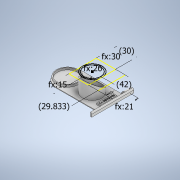
# Autodesk Inventor part: RV
Saved by Autodesk Inventor 2021 (Build 250183000, 183)
## iProperties
Created: 2020-06-05
Part Number: RV
Material: Generic
Document SubType Name: Modeling
Designer: andre
Density: 1 g/cm^3
Appearance: Default
Author: andre
## iProperties of the stored document _3DPrint.ipt
Created: 2020-06-05
Part Number: _3DPrint
Material: Generic
Document SubType Name: Modeling
Designer: andre
Density: 1 g/cm^3
Appearance: Default
Author: andre
Autodesk Inventor part; units mm, degrees
ref_plane "YZ Plane" through (0, 0, 0) normal (1, 0, 0) x (0, 1, 0)
ref_plane "XZ Plane" through (0, 0, 0) normal (0, 1, 0) x (-1, 0, 0)
ref_plane "XY Plane" through (0, 0, 0) normal (0, 0, 1) x (1, 0, 0)
sketch "Sketch1" plane through (0, 0, 0) normal (0, 1, 0) x (-1, 0, 0)
  line L0 (0, 0) -> (85, 0)
  line L1 (85, 0) -> (85, -42)
  line L2 (85, -42) -> (0, -42)
  line L3 (0, -42) -> (0, 0)
  dimension "d0" = 85
  dimension "d1" = 42
  constraints: 8 end point, 2 parallel, 1 horizontal, 1 perpendicular
  measures "d0" distance of L1.end L2.end
  measures "d1" distance of L0.end L1.end
extrude "Extrusion1" add sketch "Sketch1" along normal blind 1
sketch "Sketch2" plane through (0, 1, 0) normal (0, 1, 0) x (1, 0, 0)
  line L0 (-44.8327, 0) -> (-14.8327, 0)
  line L1 (-14.8327, 0) -> (-14.8327, 42)
  line L2 (-14.8327, 42) -> (-44.8327, 42)
  line L3 (-44.8327, 42) -> (-44.8327, 0)
  line L4 (-85, 0) -> (0, 0) projected
  dimension "d4" = 42
  dimension "d5" = 30
  dimension "d6" = 0
  constraints: 8 end point, 2 parallel, 1 horizontal, 1 perpendicular
  measures "d4" distance between parallel lines of L2 L0
  measures "d5" distance between parallel lines of L1 L3
  measures "d6" distance between parallel lines of L4 L0
extrude "Extrusion2" add sketch "Sketch2" along normal blind 28
sketch "Sketch5" plane through (0, 29, 0) normal (0, 1, 0) x (1, 0, 0)
  circle A0 centre (-29.8327, 21) radius 13
  line L0 (-44.8327, 42) -> (-44.8327, 0) projected
  line L1 (-44.8327, 0) -> (-14.8327, 0) projected
  line L2 (-14.8327, 0) -> (-14.8327, 42) projected
  line L3 (-14.8327, 42) -> (-44.8327, 42) projected
  circle A1 centre (-29.8327, 21) radius 15
  line L4 (0, 0) -> (0, 42) projected
  point P0 (-24.115, 0)
  point P1 (-44.8327, 21)
  point P2 (-14.8327, 21)
  point P3 (-19.6709, 0)
  dimension "d20" = 26
  dimension "d21" = 15
  dimension "d22" = 21
  dimension "d23" = 30
  dimension "d24" = 42
  dimension "d34" = 30
  dimension "d63" = 29.8327
  constraints: 2 centre point, 1 coincident
  measures "d20" diameter of A0
  measures "d21" distance from line of L0 A0.centre
  measures "d22" distance from line of L1 A0.centre
  measures "d23" distance between parallel lines of L2 L0
  measures "d24" distance between parallel lines of L3 L1
  measures "d34" diameter of A1
  measures "d63" distance from line of L4 A0.centre
extrude "Extrusion3" cut sketch "Sketch5" against normal blind 28 contours A0
chamfer "Chamfer3" distance 42 distance2 28 1 edges at (-29.8327, 29, -42)
extrude "Extrusion4" cut sketch "Sketch5" against normal blind 28 contours L3 L2 A1 L0 | A1 L2 L1 L0
sketch "Sketch6" plane through (0, 1, 0) normal (0, 1, 0) x (1, 0, 0)
  circle A0 centre (-68, 21) radius 15.75
  line L0 (-85, 0) -> (0, 0) projected
  circle A1 centre (-68, 21) radius 17
  line L1 (-85, 42) -> (-85, 0) projected
  point P0 (-28.5591, 0)
  dimension "d37" = 31.5
  dimension "d38" = 21
  dimension "d39" = 34
  dimension "d64" = 17
  constraints: 2 centre point, 1 coincident
  measures "d37" diameter of A0
  measures "d38" distance from line of L0 A0.centre
  measures "d39" diameter of A1
  measures "d64" distance from line of L1 A1.centre
extrude "Extrusion5" add sketch "Sketch6" along normal blind 3
fillet "Fillet3" radius 21 2 edges at (-85, 0.5, 0) (-85, 0.5, -42)
sketch "Sketch9" plane through (0, 0, 0) normal (1, 0, 0) x (0, 0, -1)
  line L0 (-11.5, 0) -> (53.5, 0)
  line L1 (53.5, 0) -> (53.5, 1)
  line L2 (53.5, 1) -> (-11.5, 1)
  line L3 (-11.5, 1) -> (-11.5, 0)
  line L4 (0, 0) -> (0, 1) projected
  dimension "d49" = 1
  dimension "d50" = 65
  dimension "d53" = 11.5
  constraints: 8 end point, 2 parallel, 1 horizontal, 1 perpendicular
  measures "d49" distance of L1.end L0.end
  measures "d50" distance between parallel lines of L1 L3
  measures "d53" distance between parallel lines of L3 L4
extrude "Extrusion8" add sketch "Sketch9" along normal blind 2
sketch "Sketch10" plane through (0, 1, 0) normal (0, 1, 0) x (1, 0, 0)
  line L0 (0, -11.5) -> (0, 0) projected
  line L1 (2, 53.5) -> (2, -11.5) projected
  line L2 (0, -11.5) -> (2, -11.5)
  line L3 (2, -11.5) -> (2, 53.5)
  line L4 (2, 53.5) -> (0, 53.5)
  line L5 (0, 53.5) -> (0, -11.5)
  point P0 (2, -11.5)
  constraints: 8 end point, 2 parallel, 1 horizontal, 1 perpendicular
extrude "Extrusion9" add sketch "Sketch10" along normal blind 5
sketch "Sketch11" plane through (0, 0, 0) normal (-1, 0, 0) x (0, 0, 1)
  line L0 (11.5, 0) -> (-53.5, 0) projected
  line L1 (-53.5, 6) -> (-42, 6)
  line L2 (-42, 6) -> (-42, 0)
  line L3 (-42, 0) -> (-53.5, 0)
  line L4 (-53.5, 0) -> (-53.5, 6)
  line L5 (-53.5, 6) -> (11.5, 6) projected
  line L6 (-53.5, 0) -> (-53.5, 6) projected
  point P0 (0, 0)
  dimension "d56" = 11.5
  dimension "d58" = 0
  dimension "d65" = 6
  constraints: 8 end point, 2 parallel, 1 horizontal, 1 perpendicular, 1 point on line
  measures "d56" distance of L2.end L3.end
  measures "d58" distance between parallel lines of L6 L4
  measures "d65" distance between parallel lines of L1 L0
extrude "Extrusion10" add sketch "Sketch11" along normal blind 6
fillet "Fillet4" radius 5.9 1 edges at (-6, 6, -47.75)
fillet "Fillet5" radius 2 1 edges at (2, 6, -21)
sketch "Sketch12" plane through (0, 1, 0) normal (0, 1, 0) x (1, 0, 0)
  line L0 (-4.5, 34) -> (-10.3327, 34)
  line L1 (-10.3327, 34) -> (-10.3327, 8)
  line L2 (-10.3327, 8) -> (-4.5, 8)
  line L3 (-4.5, 8) -> (-4.5, 34)
  line L4 (-5.931, 42) -> (-64, 42) projected
  line L5 (-64, 0) -> (0, 0) projected
  line L6 (0, 42) -> (0, -11.5) projected
  circle A0 centre (-29.8327, 21) radius 15 projected
  point P0 (0, 53.5)
  dimension "d66" = 8
  dimension "d67" = 8
  dimension "d68" = 4.5
  dimension "d69" = 4.5
  constraints: 8 end point, 2 parallel, 1 horizontal, 1 perpendicular
  measures "d66" distance between parallel lines of L4 L0
  measures "d67" distance between parallel lines of L5 L2
  measures "d68" distance between parallel lines of L6 L3
  measures "d69" distance edge to line of A0 L1
extrude "Extrusion11" add sketch "Sketch12" along normal blind 2 contours L3 L2 L1 L0
sketch "Sketch13" plane through (0, 3, 0) normal (0, 1, 0) x (1, 0, 0)
  line L0 (-4.5, 34) -> (-4.5, 8) construction
  line L1 (-4.5, 8) -> (-10.3327, 8) construction
  line L2 (-10.3327, 8) -> (-10.3327, 34) construction
  line L3 (-10.3327, 34) -> (-4.5, 34) construction
  line L4 (-4.5, 34) -> (-10.3327, 34) projected
  line L5 (-10.3327, 8) -> (-4.5, 8) projected
  line L6 (-4.5, 8) -> (-4.5, 34) projected
  line L7 (-10.3327, 34) -> (-10.3327, 8) projected
  spline S0 degree 2 poles (-8.9284, 32.2935) (-8.926, 32.1486) (-8.7618, 31.9891) (-8.6096, 31.9867) knots 0 0 0 1 2 2 2
  line L8 (-8.6096, 31.9867) -> (-7.8173, 31.9867)
  line L9 (-7.8173, 31.9867) -> (-7.8173, 31.4674)
  line L10 (-7.8173, 31.4674) -> (-8.6966, 30.9819)
  spline S1 degree 2 poles (-8.6966, 30.9819) (-8.827, 30.9118) (-8.9309, 30.7766) (-8.9284, 30.6703) knots 0 0 0 1 2 2 2
  spline S2 degree 2 poles (-8.9284, 30.6703) (-8.926, 30.535) (-8.7714, 30.3659) (-8.6482, 30.3611) knots 0 0 0 1 2 2 2
  spline S3 degree 2 poles (-8.6482, 30.3611) (-8.5975, 30.3611) (-8.5009, 30.3901) (-8.4381, 30.4263) knots 0 0 0 1 2 2 2
  line L11 (-8.4381, 30.4263) -> (-7.7086, 30.849)
  spline S4 degree 2 poles (-7.7086, 30.849) (-7.6024, 30.6051) (-7.1724, 30.3466) (-6.8946, 30.3466) knots 0 0 0 1 2 2 2
  spline S5 degree 2 poles (-6.8946, 30.3466) (-6.4574, 30.349) (-5.9695, 30.8949) (-5.9647, 31.4022) knots 0 0 0 1 2 2 2
  line L12 (-5.9647, 31.4022) -> (-5.9647, 32.2935)
  spline S6 degree 2 poles (-5.9647, 32.2935) (-5.9647, 32.4384) (-6.1313, 32.5978) (-6.2811, 32.5978) knots 0 0 0 1 2 2 2
  line L13 (-6.2811, 32.5978) -> (-8.6096, 32.5978)
  spline S7 degree 2 poles (-8.6096, 32.5978) (-8.7618, 32.5978) (-8.926, 32.4384) (-8.9284, 32.2935) knots 0 0 0 1 2 2 2
  line L14 (-7.3729, 31.9867) -> (-6.4429, 31.9867)
  line L15 (-6.4429, 31.9867) -> (-6.4429, 31.4674)
  spline S8 degree 2 poles (-6.4429, 31.4674) (-6.4453, 31.2379) (-6.6917, 30.9771) (-6.9067, 30.9746) knots 0 0 0 1 2 2 2
  spline S9 degree 2 poles (-6.9067, 30.9746) (-7.1265, 30.9746) (-7.3705, 31.2283) (-7.3729, 31.4626) knots 0 0 0 1 2 2 2
  line L16 (-7.3729, 31.4626) -> (-7.3729, 31.9867)
  spline S10 degree 2 poles (-8.9236, 29.6727) (-8.9236, 29.5447) (-8.7738, 29.4022) (-8.6386, 29.4022) knots 0 0 0 1 2 2 2
  line L17 (-8.6386, 29.4022) -> (-6.9139, 29.4022)
  line L18 (-6.9139, 29.4022) -> (-6.9139, 29.3853)
  line L19 (-6.9139, 29.3853) -> (-8.6821, 28.663)
  spline S11 degree 2 poles (-8.6821, 28.663) (-8.7763, 28.6268) (-8.8681, 28.494) (-8.8656, 28.3973) knots 0 0 0 1 2 2 2
  spline S12 degree 2 poles (-8.8656, 28.3973) (-8.8681, 28.3031) (-8.7763, 28.1751) (-8.6796, 28.1365) knots 0 0 0 1 2 2 2
  line L20 (-8.6796, 28.1365) -> (-6.9139, 27.4143)
  line L21 (-6.9139, 27.4143) -> (-6.9139, 27.3973)
  line L22 (-6.9139, 27.3973) -> (-8.6386, 27.3973)
  spline S13 degree 2 poles (-8.6386, 27.3973) (-8.7738, 27.3973) (-8.9236, 27.2572) (-8.9236, 27.1268) knots 0 0 0 1 2 2 2
  spline S14 degree 2 poles (-8.9236, 27.1268) (-8.9236, 26.9964) (-8.7738, 26.8539) (-8.6386, 26.8539) knots 0 0 0 1 2 2 2
  line L23 (-8.6386, 26.8539) -> (-6.3173, 26.8539)
  spline S15 degree 2 poles (-6.3173, 26.8539) (-6.1313, 26.8563) (-5.926, 27.0592) (-5.9236, 27.2476) knots 0 0 0 1 2 2 2
  spline S16 degree 2 poles (-5.9236, 27.2476) (-5.9236, 27.4046) (-6.0734, 27.6051) (-6.24, 27.6703) knots 0 0 0 1 2 2 2
  line L24 (-6.24, 27.6703) -> (-8.0347, 28.3925)
  line L25 (-8.0347, 28.3925) -> (-8.0347, 28.4094)
  line L26 (-8.0347, 28.4094) -> (-6.24, 29.1341)
  spline S17 degree 2 poles (-6.24, 29.1341) (-6.0709, 29.1969) (-5.9212, 29.3949) (-5.9236, 29.5519) knots 0 0 0 1 2 2 2
  spline S18 degree 2 poles (-5.9236, 29.5519) (-5.926, 29.7403) (-6.1313, 29.9457) (-6.3173, 29.9457) knots 0 0 0 1 2 2 2
  line L27 (-6.3173, 29.9457) -> (-8.6386, 29.9457)
  spline S19 degree 2 poles (-8.6386, 29.9457) (-8.7738, 29.9457) (-8.9236, 29.8031) (-8.9236, 29.6727) knots 0 0 0 1 2 2 2
  line L28 (-8.885, 25.2452) -> (-8.885, 24.2572)
  spline S20 degree 2 poles (-8.885, 24.2572) (-8.8801, 23.7838) (-8.4381, 23.2524) (-8.0492, 23.2476) knots 0 0 0 1 2 2 2
  spline S21 degree 2 poles (-8.0492, 23.2476) (-7.7545, 23.2524) (-7.3705, 23.6316) (-7.3415, 23.936) knots 0 0 0 1 2 2 2
  line L29 (-7.3415, 23.936) -> (-7.327, 23.936)
  spline S22 degree 2 poles (-7.327, 23.936) (-7.2859, 23.6969) (-6.9381, 23.3925) (-6.6917, 23.3877) knots 0 0 0 1 2 2 2
  spline S23 degree 2 poles (-6.6917, 23.3877) (-6.3536, 23.3901) (-5.9671, 23.8635) (-5.9647, 24.279) knots 0 0 0 1 2 2 2
  line L30 (-5.9647, 24.279) -> (-5.9647, 25.2452)
  spline S24 degree 2 poles (-5.9647, 25.2452) (-5.9647, 25.3901) (-6.1313, 25.5495) (-6.2811, 25.5495) knots 0 0 0 1 2 2 2
  line L31 (-6.2811, 25.5495) -> (-8.5661, 25.5495)
  spline S25 degree 2 poles (-8.5661, 25.5495) (-8.7183, 25.5495) (-8.885, 25.3901) (-8.885, 25.2452) knots 0 0 0 1 2 2 2
  line L32 (-8.4284, 24.9384) -> (-7.5806, 24.9384)
  line L33 (-7.5806, 24.9384) -> (-7.5806, 24.4263)
  spline S26 degree 2 poles (-7.5806, 24.4263) (-7.583, 24.1558) (-7.7956, 23.8708) (-8.0009, 23.8708) knots 0 0 0 1 2 2 2
  spline S27 degree 2 poles (-8.0009, 23.8708) (-8.211, 23.8708) (-8.4284, 24.1486) (-8.4284, 24.4143) knots 0 0 0 1 2 2 2
  line L34 (-8.4284, 24.4143) -> (-8.4284, 24.9384)
  line L35 (-7.1796, 24.9384) -> (-6.4188, 24.9384)
  line L36 (-6.4188, 24.9384) -> (-6.4188, 24.4384)
  spline S28 degree 2 poles (-6.4188, 24.4384) (-6.4212, 24.221) (-6.612, 23.9891) (-6.7883, 23.9891) knots 0 0 0 1 2 2 2
  spline S29 degree 2 poles (-6.7883, 23.9891) (-6.9743, 23.9891) (-7.1772, 24.2548) (-7.1796, 24.5012) knots 0 0 0 1 2 2 2
  line L37 (-7.1796, 24.5012) -> (-7.1796, 24.9384)
  spline S30 degree 2 poles (-8.9236, 22.7041) (-8.9236, 22.5833) (-8.7932, 22.436) (-8.6482, 22.3949) knots 0 0 0 1 2 2 2
  line L38 (-8.6482, 22.3949) -> (-8.1917, 22.2403)
  line L39 (-8.1917, 22.2403) -> (-8.1917, 21.1872)
  line L40 (-8.1917, 21.1872) -> (-8.6531, 21.0326)
  spline S31 degree 2 poles (-8.6531, 21.0326) (-8.7956, 20.9915) (-8.9236, 20.8418) (-8.9236, 20.7138) knots 0 0 0 1 2 2 2
  spline S32 degree 2 poles (-8.9236, 20.7138) (-8.9212, 20.5785) (-8.7642, 20.4118) (-8.6362, 20.4094) knots 0 0 0 1 2 2 2
  spline S33 degree 2 poles (-8.6362, 20.4094) (-8.5903, 20.4094) (-8.5009, 20.4263) (-8.4405, 20.4481) knots 0 0 0 1 2 2 2
  line L41 (-8.4405, 20.4481) -> (-6.269, 21.25)
  spline S34 degree 2 poles (-6.269, 21.25) (-6.0903, 21.3128) (-5.9236, 21.5374) (-5.9236, 21.7162) knots 0 0 0 1 2 2 2
  spline S35 degree 2 poles (-5.9236, 21.7162) (-5.9236, 21.8877) (-6.0927, 22.1123) (-6.269, 22.1751) knots 0 0 0 1 2 2 2
  line L42 (-6.269, 22.1751) -> (-8.4405, 22.9722)
  spline S36 degree 2 poles (-8.4405, 22.9722) (-8.4985, 22.994) (-8.5975, 23.0133) (-8.6362, 23.0133) knots 0 0 0 1 2 2 2
  spline S37 degree 2 poles (-8.6362, 23.0133) (-8.769, 23.0133) (-8.9212, 22.849) (-8.9236, 22.7041) knots 0 0 0 1 2 2 2
  line L43 (-7.7183, 22.1075) -> (-6.5226, 21.7283)
  line L44 (-6.5226, 21.7283) -> (-6.5226, 21.7138)
  line L45 (-6.5226, 21.7138) -> (-7.7183, 21.3273)
  line L46 (-7.7183, 21.3273) -> (-7.7183, 22.1075)
  spline S38 degree 2 poles (-8.9333, 18.9698) (-8.9284, 18.4191) (-8.4357, 17.7983) (-8.0033, 17.7935) knots 0 0 0 1 2 2 2
  spline S39 degree 2 poles (-8.0033, 17.7935) (-7.6724, 17.7911) (-7.2763, 18.2186) (-7.1869, 18.68) knots 0 0 0 1 2 2 2
  line L47 (-7.1869, 18.68) -> (-7.1241, 18.9891)
  spline S40 degree 2 poles (-7.1241, 18.9891) (-7.0734, 19.2452) (-6.897, 19.4771) (-6.7642, 19.4746) knots 0 0 0 1 2 2 2
  spline S41 degree 2 poles (-6.7642, 19.4746) (-6.5999, 19.4698) (-6.4091, 19.2017) (-6.4067, 18.9722) knots 0 0 0 1 2 2 2
  spline S42 degree 2 poles (-6.4067, 18.9722) (-6.4067, 18.7838) (-6.554, 18.5085) (-6.7183, 18.436) knots 0 0 0 1 2 2 2
  spline S43 degree 2 poles (-6.7183, 18.436) (-6.8125, 18.3853) (-6.8995, 18.2452) (-6.8995, 18.1437) knots 0 0 0 1 2 2 2
  spline S44 degree 2 poles (-6.8995, 18.1437) (-6.897, 18.0254) (-6.7642, 17.8853) (-6.6555, 17.8829) knots 0 0 0 1 2 2 2
  spline S45 degree 2 poles (-6.6555, 17.8829) (-6.6144, 17.8829) (-6.5492, 17.8949) (-6.5178, 17.9046) knots 0 0 0 1 2 2 2
  spline S46 degree 2 poles (-6.5178, 17.9046) (-6.2304, 18.006) (-5.9164, 18.5664) (-5.9139, 18.9722) knots 0 0 0 1 2 2 2
  spline S47 degree 2 poles (-5.9139, 18.9722) (-5.9164, 19.2983) (-6.1362, 19.8007) (-6.5323, 20.0833) (-6.8028, 20.0882) knots 0 0 0 1 2 3 3 3
  spline S48 degree 2 poles (-6.8028, 20.0882) (-7.1289, 20.0882) (-7.5444, 19.6558) (-7.6313, 19.2186) knots 0 0 0 1 2 2 2
  line L48 (-7.6313, 19.2186) -> (-7.6917, 18.9094)
  spline S49 degree 2 poles (-7.6917, 18.9094) (-7.7473, 18.6365) (-7.926, 18.4022) (-8.0685, 18.4046) knots 0 0 0 1 2 2 2
  spline S50 degree 2 poles (-8.0685, 18.4046) (-8.2328, 18.4094) (-8.4381, 18.7065) (-8.4405, 18.9553) knots 0 0 0 1 2 2 2
  spline S51 degree 2 poles (-8.4405, 18.9553) (-8.4429, 19.1679) (-8.2835, 19.4843) (-8.1168, 19.5592) knots 0 0 0 1 2 2 2
  spline S52 degree 2 poles (-8.1168, 19.5592) (-8.0226, 19.6123) (-7.9381, 19.7476) (-7.9405, 19.8394) knots 0 0 0 1 2 2 2
  spline S53 degree 2 poles (-7.9405, 19.8394) (-7.9405, 19.9601) (-8.0854, 20.1075) (-8.2086, 20.1099) knots 0 0 0 1 2 2 2
  spline S54 degree 2 poles (-8.2086, 20.1099) (-8.2497, 20.1099) (-8.3342, 20.093) (-8.3729, 20.0761) knots 0 0 0 1 2 2 2
  spline S55 degree 2 poles (-8.3729, 20.0761) (-8.6168, 19.9867) (-8.9284, 19.4239) (-8.9333, 18.9698) knots 0 0 0 1 2 2 2
  line L49 (-8.885, 17.1171) -> (-8.885, 15.7283)
  spline S56 degree 2 poles (-8.885, 15.7283) (-8.885, 15.6002) (-8.7521, 15.4529) (-8.6313, 15.4505) knots 0 0 0 1 2 2 2
  spline S57 degree 2 poles (-8.6313, 15.4505) (-8.513, 15.4529) (-8.3801, 15.6027) (-8.3801, 15.7283) knots 0 0 0 1 2 2 2
  line L50 (-8.3801, 15.7283) -> (-8.3801, 16.8104)
  line L51 (-8.3801, 16.8104) -> (-7.641, 16.8104)
  line L52 (-7.641, 16.8104) -> (-7.641, 15.7814)
  spline S58 degree 2 poles (-7.641, 15.7814) (-7.641, 15.663) (-7.5178, 15.5278) (-7.4067, 15.5254) knots 0 0 0 1 2 2 2
  spline S59 degree 2 poles (-7.4067, 15.5254) (-7.298, 15.5278) (-7.1724, 15.6655) (-7.1724, 15.7814) knots 0 0 0 1 2 2 2
  line L53 (-7.1724, 15.7814) -> (-7.1724, 16.8104)
  line L54 (-7.1724, 16.8104) -> (-6.4695, 16.8104)
  line L55 (-6.4695, 16.8104) -> (-6.4695, 15.7283)
  spline S60 degree 2 poles (-6.4695, 15.7283) (-6.4695, 15.6027) (-6.3367, 15.4529) (-6.2183, 15.4505) knots 0 0 0 1 2 2 2
  spline S61 degree 2 poles (-6.2183, 15.4505) (-6.0975, 15.4529) (-5.9647, 15.6002) (-5.9647, 15.7283) knots 0 0 0 1 2 2 2
  line L56 (-5.9647, 15.7283) -> (-5.9647, 17.1171)
  spline S62 degree 2 poles (-5.9647, 17.1171) (-5.9647, 17.2621) (-6.1313, 17.4215) (-6.2811, 17.4215) knots 0 0 0 1 2 2 2
  line L57 (-6.2811, 17.4215) -> (-8.5661, 17.4215)
  spline S63 degree 2 poles (-8.5661, 17.4215) (-8.7183, 17.4215) (-8.885, 17.2621) (-8.885, 17.1171) knots 0 0 0 1 2 2 2
  spline S64 degree 2 poles (-8.9236, 13.064) (-8.9236, 12.8877) (-8.7545, 12.663) (-8.5709, 12.5978) knots 0 0 0 1 2 2 2
  line L58 (-8.5709, 12.5978) -> (-6.3681, 11.779)
  spline S65 degree 2 poles (-6.3681, 11.779) (-6.2859, 11.75) (-6.2062, 11.75) knots 0 0 0 1 1 1
  spline S66 degree 2 poles (-6.2062, 11.75) (-6.0782, 11.7524) (-5.926, 11.9215) (-5.9236, 12.064) knots 0 0 0 1 2 2 2
  spline S67 degree 2 poles (-5.9236, 12.064) (-5.9236, 12.1824) (-6.0371, 12.3273) (-6.1579, 12.3659) knots 0 0 0 1 2 2 2
  line L59 (-6.1579, 12.3659) -> (-8.2545, 13.0471)
  line L60 (-8.2545, 13.0471) -> (-8.2545, 13.0616)
  line L61 (-8.2545, 13.0616) -> (-6.1652, 13.7452)
  spline S68 degree 2 poles (-6.1652, 13.7452) (-6.0395, 13.7814) (-5.9236, 13.9336) (-5.9236, 14.0568) knots 0 0 0 1 2 2 2
  spline S69 degree 2 poles (-5.9236, 14.0568) (-5.926, 14.2041) (-6.083, 14.3756) (-6.2135, 14.378) knots 0 0 0 1 2 2 2
  spline S70 degree 2 poles (-6.2135, 14.378) (-6.3004, 14.378) (-6.385, 14.349) knots 0 0 0 1 1 1
  line L62 (-6.385, 14.349) -> (-8.5685, 13.535)
  spline S71 degree 2 poles (-8.5685, 13.535) (-8.7545, 13.4698) (-8.9236, 13.2428) (-8.9236, 13.064) knots 0 0 0 1 2 2 2
  line L63 (-8.885, 11.1679) -> (-8.885, 9.5519)
  spline S72 degree 2 poles (-8.885, 9.5519) (-8.8825, 9.4312) (-8.7521, 9.2983) (-8.641, 9.2983) knots 0 0 0 1 2 2 2
  spline S73 degree 2 poles (-8.641, 9.2983) (-8.5299, 9.2983) (-8.3995, 9.4312) (-8.3995, 9.5519) knots 0 0 0 1 2 2 2
  line L64 (-8.3995, 9.5519) -> (-8.3995, 10.6534)
  line L65 (-8.3995, 10.6534) -> (-8.3874, 10.6534)
  line L66 (-8.3874, 10.6534) -> (-7.7787, 10.0205)
  spline S74 degree 2 poles (-7.7787, 10.0205) (-7.5565, 9.7838) (-7.2255, 9.4964) (-6.9236, 9.3684) (-6.7497, 9.3684) knots 0 0 0 1 2 3 3 3
  spline S75 degree 2 poles (-6.7497, 9.3684) (-6.4961, 9.3708) (-6.1144, 9.6292) (-5.9019, 10.093) (-5.8995, 10.4046) knots 0 0 0 1 2 3 3 3
  spline S76 degree 2 poles (-5.8995, 10.4046) (-5.9019, 10.6824) (-6.0782, 11.1027) (-6.3608, 11.3732) (-6.5251, 11.4239) knots 0 0 0 1 2 3 3 3
  spline S77 degree 2 poles (-6.5251, 11.4239) (-6.5565, 11.4336) (-6.6217, 11.4457) (-6.6555, 11.4457) knots 0 0 0 1 2 2 2
  spline S78 degree 2 poles (-6.6555, 11.4457) (-6.7714, 11.4457) (-6.9043, 11.308) (-6.9043, 11.1848) knots 0 0 0 1 2 2 2
  spline S79 degree 2 poles (-6.9043, 11.1848) (-6.9067, 11.0882) (-6.8173, 10.9626) (-6.728, 10.9143) knots 0 0 0 1 2 2 2
  spline S80 degree 2 poles (-6.728, 10.9143) (-6.5516, 10.8345) (-6.3753, 10.5882) (-6.3753, 10.4118) knots 0 0 0 1 2 2 2
  spline S81 degree 2 poles (-6.3753, 10.4118) (-6.3777, 10.2114) (-6.6048, 9.9674) (-6.7883, 9.965) knots 0 0 0 1 2 2 2
  spline S82 degree 2 poles (-6.7883, 9.965) (-6.8898, 9.9626) (-7.0806, 10.0399) (-7.3149, 10.2379) (-7.4864, 10.4167) knots 0 0 0 1 2 3 3 3
  line L67 (-7.4864, 10.4167) -> (-8.3173, 11.2886)
  spline S83 degree 2 poles (-8.3173, 11.2886) (-8.4019, 11.3804) (-8.5395, 11.4577) (-8.6241, 11.4553) knots 0 0 0 1 2 2 2
  spline S84 degree 2 poles (-8.6241, 11.4553) (-8.74, 11.4553) (-8.8825, 11.3128) (-8.885, 11.1679) knots 0 0 0 1 2 2 2
  point P0 (0, 0)
  dimension "d72" = 0
  dimension "d73" = 0
  dimension "d74" = 0
  dimension "d75" = 0
  constraints: 2 other
  measures "d72" distance between parallel lines of L4 L3
  measures "d73" distance between parallel lines of L5 L1
  measures "d74" distance between parallel lines of L6 L0
  measures "d75" distance between parallel lines of L7 L2
extrude "Extrusion12" cut sketch "Sketch13" against normal blind 2 contours S7 L13 S6 L12 S5 S4 L11 S3 S2 S1 L10 L9 L8 S0 | S19 L27 S18 S17 L26 L25 L24 S16 S15 L23 S14 S13 L22 L21 L20 S12 S11 L19 L18 L17 S10 | S25 L31 S24 L30 S23 S22 L29 S21 S20 L28 | S37 S36 L42 S35 S34 L41 S33 S32 S31 L40 L39 L38 S30 | S55 S54 S53 S52 S51 S50 S49 L48 S48 S47 S46 S45 S44 S43 S42 S41 S40 L47 S39 S38 | S63 L57 S62 L56 S61 S60 L55 L54 L53 S59 S58 L52 L51 L50 S57 S56 L49 | S71 L62 S70 S69 S68 L61 L60 L59 S67 S66 S65 L58 S64 | S84 S83 L67 S82 S81 S80 S79 S78 S77 S76 S75 S74 L66 L65 L64 S73 S72 L63
equation "\"d4\" = d1"
equation "\"d21\" = 0.5 * d23"
equation "\"d22\" = 0.5 * d1"
equation "\"d34\" = d23"
equation "\"d25\" = d7"
equation "\"d30\" = d1"
equation "\"d31\" = d7"
equation "\"d38\" = 0.5 * d1"
equation "\"d64\" = 0.5 * d39"
equation "\"d42\" = 0.5 * d1"
equation "\"d53\" = -0.5 * d1 + 0.5 * d50"
equation "\"d56\" = d53"
equation "\"d67\" = d66"
equation "\"d69\" = d68"
equation "\"d7\" = 28"
body "Solid1"
